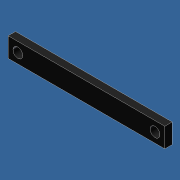
# Autodesk Inventor part: GE-12024
Saved by Autodesk Inventor 2012 (Build 160160000, 160)
## iProperties
Created: 2011-06-15
Part Number: GE-12024
Document SubType Name: Modeling
Designer: dfoster
Density: 1 g/cm^3
Description: Hinge Plate, Double
Mass: 47.3713 g
Surface Area: 149.989 cm^2
Volume: 47.3713 cm^3
Material: Default
Title: Hinge Plate, Double
Author: dfoster
Autodesk Inventor part; units mm, degrees
ref_plane "YZ Plane" through (0, 0, 0) normal (1, 0, 0) x (0, 1, 0)
ref_plane "XZ Plane" through (0, 0, 0) normal (0, 1, 0) x (-1, 0, 0)
ref_plane "XY Plane" through (0, 0, 0) normal (0, 0, 1) x (1, 0, 0)
sketch "Sketch1" plane through (0, 0, 0) normal (0, 0, 1) x (1, 0, 0)
  line L0 (0, 0) -> (203.2, 0)
  line L1 (203.2, 0) -> (203.2, 25.4)
  line L2 (203.2, 25.4) -> (0, 25.4)
  line L3 (0, 25.4) -> (0, 0)
  circle A0 centre (12.7, 12.7) radius 6.35
  circle A1 centre (190.5, 12.7) radius 6.35
  dimension "d0" = 203.2
  dimension "d1" = 25.4
  dimension "d2" = 12.7
  dimension "d3" = 12.7
  dimension "d4" = 12.7
  dimension "d5" = 12.7
  dimension "d9" = 12.7
  dimension "d10" = 12.7
  constraints: 8 end point, 2 centre point, 2 parallel, 1 horizontal, 1 perpendicular
  measures "d0" distance of L1.end L2.end
  measures "d1" distance between parallel lines of L0 L2
  measures "d2" distance from line of A0.centre L2
  measures "d3" distance from line of A1.centre L2
  measures "d4" distance from line of A0.centre L3
  measures "d5" distance from line of A1.centre L1
  measures "d9" diameter of A0
  measures "d10" diameter of A1
extrude "Extrusion1" add sketch "Sketch1" along normal blind 9.652
equation "\"d2\" = 0.5 * d1"
equation "\"d3\" = d2"
equation "\"d4\" = d2"
equation "\"d5\" = d3"
body "Solid1"
